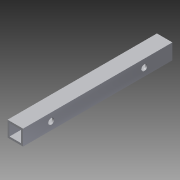
# Autodesk Inventor part: box alluminum custom 6in
Saved by Autodesk Inventor 2013 (Build 170138000, 138)
## iProperties
Created: 2013-12-23
Part Number: box alluminum custom 6in
Material: Aluminum 6061
Document SubType Name: Modeling
Designer: kahohbein
Density: 1 g/cm^3
Author: kahohbein
Autodesk Inventor part; units mm, degrees
ref_plane "YZ Plane" through (0, 0, 0) normal (1, 0, 0) x (0, 1, 0)
ref_plane "XZ Plane" through (0, 0, 0) normal (0, 1, 0) x (-1, 0, 0)
ref_plane "XY Plane" through (0, 0, 0) normal (0, 0, 1) x (1, 0, 0)
sketch "Sketch1" plane through (0, 0, 0) normal (0, 0, 1) x (1, 0, 0)
  line L0 (-6.35, -6.35) -> (6.35, -6.35)
  line L1 (6.35, -6.35) -> (6.35, 6.35)
  line L2 (6.35, 6.35) -> (-6.35, 6.35)
  line L3 (-6.35, 6.35) -> (-6.35, -6.35)
  line L4 (-6.35, -6.35) -> (6.35, 6.35) construction
  line L5 (6.35, -6.35) -> (-6.35, 6.35) construction
  line L6 (-4.7625, -4.7625) -> (4.7625, -4.7625)
  line L7 (4.7625, -4.7625) -> (4.7625, 4.7625)
  line L8 (4.7625, 4.7625) -> (-4.7625, 4.7625)
  line L9 (-4.7625, 4.7625) -> (-4.7625, -4.7625)
  line L10 (-4.7625, -4.7625) -> (4.7625, 4.7625) construction
  line L11 (4.7625, -4.7625) -> (-4.7625, 4.7625) construction
  point P0 (0, 0)
  dimension "d0" = 12.7
  dimension "d1" = 12.7
  dimension "d2" = 9.525
  dimension "d3" = 9.525
  constraints: 24 end point, 4 midpoint, 4 parallel, 2 horizontal, 2 perpendicular
  measures "d0" distance of L2.end L1.end
  measures "d1" distance of L1.end L0.end
  measures "d2" distance of L8.end L7.end
  measures "d3" distance of L7.end L6.end
extrude "Extrusion1" add sketch "Sketch1" along normal blind 160.3375
sketch "Sketch2" plane through (6.35, -6.35, 0) normal (1, 0, 0) x (0, 0, -1)
  circle A0 centre (-118.2688, 6.35) radius 2.413
  circle A1 centre (-42.0688, 6.35) radius 2.413
  line L0 (0, 0) -> (0, 12.7) projected
  line L1 (-160.3375, 0) -> (-160.3375, 12.7) projected
  line L2 (0, 0) -> (-160.3375, 0) projected
  line L3 (-118.2688, 6.35) -> (-42.0688, 6.35)
  line L4 (-118.2688, 6.35) -> (-160.3375, 6.35)
  line L5 (-42.0688, 6.35) -> (0, 6.35)
  dimension "d6" = 4.826
  dimension "d7" = 4.826
  dimension "d10" = 76.2
  constraints: 6 end point, 2 centre point, 1 collinear, 1 midpoint, 1 parallel, 1 perpendicular
  measures "d6" diameter of A0
  measures "d7" diameter of A1
  measures "d10" distance of L3.start L3.end
extrude "Extrusion2" cut sketch "Sketch2" against normal blind 160.3375 contours L3 L4 A0 | A0 L4 L3 | L3 L5 A1 | A1 L5 L3
sketch "Sketch3" plane through (6.35, -6.35, 0) normal (1, 0, 0) x (0, 0, -1)
  line L0 (-160.3375, 0) -> (-160.3375, 12.7) projected
  line L1 (-179.3875, -12.1882) -> (-141.2875, -12.1882)
  line L2 (-141.2875, -12.1882) -> (-141.2875, 24.8882)
  line L3 (-141.2875, 24.8882) -> (-179.3875, 24.8882)
  line L4 (-179.3875, 24.8882) -> (-179.3875, -12.1882)
  line L5 (-179.3875, -12.1882) -> (-141.2875, 24.8882) construction
  line L6 (-141.2875, -12.1882) -> (-179.3875, 24.8882) construction
  line L7 (-19.05, -6.325) -> (19.05, -6.325)
  line L8 (19.05, -6.325) -> (19.05, 19.025)
  line L9 (19.05, 19.025) -> (-19.05, 19.025)
  line L10 (-19.05, 19.025) -> (-19.05, -6.325)
  line L11 (-19.05, -6.325) -> (19.05, 19.025) construction
  line L12 (19.05, -6.325) -> (-19.05, 19.025) construction
  point P0 (0, 6.35)
  point P1 (-160.3375, 6.35)
  dimension "d11" = 38.1
  dimension "d12" = 38.1
  constraints: 24 end point, 5 midpoint, 4 parallel, 2 horizontal, 2 perpendicular
  measures "d11" distance of L3.end L2.end
  measures "d12" distance of L9.end L8.end
extrude "Extrusion3" cut sketch "Sketch3" against normal blind 160.3375
body "Solid1"
